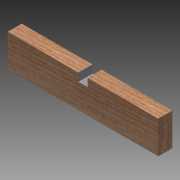
# Autodesk Inventor part: CNC_1.1v_X_1(faceplate)
Saved by Autodesk Inventor 2015 (Build 190159000, 159)
## iProperties
Created: 2015-07-10
Part Number: CNC_1.1v_X_1(faceplate)
Material: Generic
Document SubType Name: Modeling
Designer: Bangladesh
Density: 1 g/cm^3
Appearance: Default
Author: Bangladesh
Autodesk Inventor part; units mm, degrees
ref_plane "YZ Plane" through (0, 0, 0) normal (1, 0, 0) x (0, 1, 0)
ref_plane "XZ Plane" through (0, 0, 0) normal (0, 1, 0) x (-1, 0, 0)
ref_plane "XY Plane" through (0, 0, 0) normal (0, 0, 1) x (1, 0, 0)
sketch "Sketch1" plane through (0, 0, 0) normal (1, 0, 0) x (0, 1, 0)
  line L0 (44.45, 19.05) -> (-44.45, 19.05)
  line L1 (-44.45, 19.05) -> (-44.45, -19.05)
  line L2 (-44.45, -19.05) -> (44.45, -19.05)
  line L3 (44.45, -19.05) -> (44.45, 19.05)
  line L4 (44.45, 19.05) -> (-44.45, -19.05) construction
  line L5 (-44.45, 19.05) -> (44.45, -19.05) construction
  point P0 (0, 0)
  dimension "d0" = 88.9
  dimension "d1" = 38.1
  constraints: 12 end point, 2 midpoint, 2 parallel, 1 horizontal, 1 perpendicular
  measures "d0" distance of L2.end L1.end
  measures "d1" distance of L1.end L0.end
extrude "Extrusion1" add sketch "Sketch1" along normal mid plane 410
sketch "Sketch2" plane through (-205, -44.45, 19.05) normal (0, 0, 1) x (1, 0, 0)
  line L0 (0, 88.9) -> (0, 0) projected
  line L1 (0, 67.1803) -> (192.497, 67.1803)
  line L2 (0, 88.9) -> (410, 88.9) projected
  line L3 (192.497, 88.9) -> (192.497, 67.1803)
  line L4 (192.497, 67.1803) -> (217.497, 67.1803)
  line L5 (217.497, 67.1803) -> (217.497, 88.9)
  point P0 (205, 44.45)
  dimension "d14" = 192.497
  dimension "d15" = 25
  constraints: 8 end point, 3 point on line, 2 horizontal, 2 perpendicular
  measures "d14" distance of L1.start L1.end
  measures "d15" distance of L1.end L4.end
extrude "Extrusion2" cut sketch "Sketch2" against normal blind 166.2125 contours L2 L5 L4 L3
body "Solid1"
